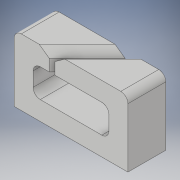
# Autodesk Inventor part: Cable Clip v1
Saved by Autodesk Inventor 2019 (Build 230136000, 136)
## iProperties
Created: 2021-08-22
Part Number: Cable Clip v1
Material: Generic
Document SubType Name: Modeling
Designer: Lix
Density: 1 g/cm^3
Appearance: Default
Author: Lix
Autodesk Inventor part; units mm, degrees
ref_plane "YZ Plane" through (0, 0, 0) normal (1, 0, 0) x (0, 1, 0)
ref_plane "XZ Plane" through (0, 0, 0) normal (0, 1, 0) x (-1, 0, 0)
ref_plane "XY Plane" through (0, 0, 0) normal (0, 0, 1) x (1, 0, 0)
sketch "Sketch1" plane through (0, 0, 0) normal (0, 0, 1) x (1, 0, 0)
  circle A0 centre (0, 0) radius 1 construction
  circle A1 centre (2.5, 0) radius 1 construction
  circle A2 centre (-2.5, 0) radius 1 construction
  circle A3 centre (-1.25, 2) radius 1 construction
  circle A4 centre (1.25, 2) radius 1 construction
  line L0 (-4, 2.5) -> (4, 2.5)
  line L1 (4, 2.5) -> (4, -0.5)
  line L2 (4, -0.5) -> (-4, -0.5)
  line L3 (-4, -0.5) -> (-4, 2.5)
  line L4 (-4, 2.5) -> (4, -0.5) construction
  line L5 (4, 2.5) -> (-4, -0.5) construction
  line L6 (6, 4.5) -> (-6, 4.5)
  line L7 (-6, 4.5) -> (-6, -2.5)
  line L8 (-6, -2.5) -> (6, -2.5)
  line L9 (6, -2.5) -> (6, 4.5)
  point P0 (0, 1)
  point P1 (0, 1)
  dimension "d0" = 2
  dimension "d1" = 2.5
  dimension "d2" = 2.5
  dimension "d3" = 1.25
  dimension "d4" = 2
  dimension "d5" = 1.25
  dimension "d6" = 1
  dimension "d7" = 3
  dimension "d8" = 8
  dimension "d9" = 2
  constraints: 20 end point, 5 centre point, 4 equal radius, 4 parallel, 3 midpoint, 2 perpendicular, 1 coincident, 1 horizontal, 1 horizontal alignment, 1 vertical alignment, 3 other
  measures "d0" diameter of A0
  measures "d1" distance of A2.centre point (0, 0)
  measures "d2" distance of A1.centre point (0, 0)
  measures "d3" horizontal distance of point (0, 0) A3.centre
  measures "d4" vertical distance of A3.centre point (0, 0)
  measures "d5" horizontal distance of A4.centre point (0, 0)
  measures "d6" distance of point (0, 1) point (0, 0)
  measures "d7" distance of L0.end L1.end
  measures "d8" distance of L0.start L0.end
  measures "d9" distance between parallel lines of L0 L6
extrude "Extrusion1" add sketch "Sketch1" along normal blind 4
sketch "Sketch2" plane through (-6, 4.5, 0) normal (0, 1, 0) x (1, 0, 0)
  line L0 (2, 0) -> (2, -4) projected
  line L1 (10, 0) -> (10, -4) projected
  line L2 (4, -4) -> (8, 0) construction
  line L3 (12, -4) -> (0, -4) projected
  line L4 (12, 0) -> (0, 0) projected
  line L5 (3.7, -4) -> (7.7, 0)
  line L6 (10, 0) -> (2, 0) projected
  line L7 (4.3, -4) -> (8.3, 0)
  line L8 (3.7, -4) -> (4.3, -4)
  line L9 (7.7, 0) -> (8.3, 0)
  point P0 (6, 0)
  dimension "d12" = 2
  dimension "d13" = 2
  dimension "d15" = 0.3
  dimension "d16" = 0.3
  constraints: 10 end point, 6 point on line, 2 collinear, 2 parallel
  measures "d12" distance of L2.start L0.end
  measures "d13" distance of L1.start L2.end
  measures "d15" distance of L5.start L2.start
  measures "d16" distance of L7.start L2.start
extrude "Extrusion2" cut sketch "Sketch2" against normal blind 4 contours L4 L7 L3 L5
chamfer "Chamfer1" distance 0.75 angle 45 2 edges at (0.3, 4.5, 2) (-0.3, 4.5, 2)
fillet "Fillet1" radius 0.75 4 edges at (-4, -0.5, 2) (-4, 2.5, 2) (4, 2.5, 2) (4, -0.5, 2)
fillet "Fillet1" radius 0.75 2 edges at (-6, 4.5, 2) (6, 4.5, 2)
equation "\"d2\" = d1"
equation "\"d5\" = d3"
equation "\"d13\" = d12"
equation "\"d16\" = d15"
body "Solid1"
